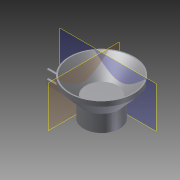
# Autodesk Inventor part: BallReciever
Saved by Autodesk Inventor 2012 (Build 160160000, 160)
## iProperties
Created: 2013-07-09
Part Number: BallReciever
Material: Default
Document SubType Name: Modeling
Designer: 1
Density: 1 g/cm^3
Author: 1
Autodesk Inventor part; units mm, degrees
ref_plane "XZ Plane" through (0, 0, 0) normal (0, 1, 0) x (-1, 0, 0)
ref_plane "XY Plane" through (0, 0, 0) normal (0, 0, 1) x (1, 0, 0)
sketch "Sketch1" plane through (0, 0, 0) normal (0, 0, 1) x (1, 0, 0)
  line L0 (34, 31.2954) -> (15.654, 31.2954)
  line L1 (15.654, 31.2954) -> (15.654, 48.2362)
  line L2 (15.654, 48.2362) -> (1.0463, 64.8622)
  line L3 (1.0463, 64.8622) -> (1.0463, 69.6686)
  line L4 (1.0463, 69.6686) -> (2.3392, 69.6686)
  line L5 (2.3392, 69.6686) -> (17.6799, 52.2084)
  line L6 (17.6799, 52.2084) -> (34, 52.2084)
  line L7 (52, 820) -> (16, 820) projected
  line L8 (34, 820) -> (34, 0)
  point P0 (0, 0)
  constraints: 16 end point, 3 parallel, 3 perpendicular, 2 point on line, 1 midpoint
revolve "Revolution1" add sketch "Sketch1" angle 360 about axis through (34, 820, 0) along (0, -1, 0)
ref_plane "Work Plane1" through (15.654, 39.7658, 0) normal (1, 0, 0) x (0, 1, 0)
sketch "Sketch2" plane through (15.654, 39.7658, 0) normal (1, 0, 0) x (0, 1, 0)
  line L0 (-8.4704, -18.346) -> (-8.4704, 18.346) construction
  line L1 (-2.4704, -2.5) -> (-7.4704, -2.5)
  line L2 (-7.4704, -2.5) -> (-7.4704, -0.5)
  line L3 (-7.4704, -0.5) -> (-2.4704, -0.5)
  line L4 (-2.4704, -0.5) -> (-2.4704, -2.5)
  line L5 (6.5296, -2.5) -> (1.5296, -2.5)
  line L6 (1.5296, -2.5) -> (1.5296, -0.5)
  line L7 (1.5296, -0.5) -> (6.5296, -0.5)
  line L8 (6.5296, -0.5) -> (6.5296, -2.5)
  line L9 (6.5296, -2.5) -> (1.5296, -0.5) construction
  line L10 (6.5296, -0.5) -> (1.5296, -2.5) construction
  line L11 (-7.4704, -0.5) -> (-2.4704, -2.5) construction
  line L12 (-7.4704, -2.5) -> (-2.4704, -0.5) construction
  line L13 (-39.7658, 0) -> (810.2342, 0) projected
  dimension "d1" = 5
  dimension "d2" = 2
  dimension "d3" = 1
  dimension "d4" = 4
  dimension "d10" = 0.5
  constraints: 24 end point, 4 parallel, 2 equal length, 2 horizontal, 2 perpendicular, 1 collinear
  measures "d1" distance of L5.start L5.end
  measures "d2" distance of L7.end L5.start
  measures "d3" distance between parallel lines of L0 L2
  measures "d4" distance between parallel lines of L6 L4
  measures "d10" distance between parallel lines of L7 L13
extrude "Extrusion1" add sketch "Sketch2" along normal blind 2.0625 and the other way blind 38.3375
ref_plane "Work Plane3" through (34, 39.7658, -18.346) normal (0, 0, -1) x (-1, 0, 0)
ref_plane "Work Plane2" through (-80, 0, -3) normal (0, 0, -1) x (-1, 0, 0)
sketch "Sketch3" plane through (34, 39.7658, -18.346) normal (0, 0, -1) x (-1, 0, 0)
  circle A0 centre (0, 0) radius 2.5
  circle A1 centre (0, 779.9029) radius 2.5 projected
  point P0 (34, -39.7658)
  constraints: 1 centre point, 1 equal radius
extrude "Extrusion2" add sketch "Sketch3" along normal blind 11.5875 and the other way blind 5.7935 contours A0
body "Solid1"
